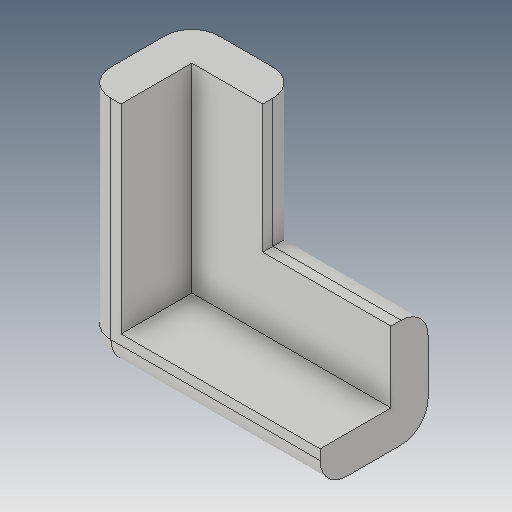
# Autodesk Inventor part: クッション
Saved by Autodesk Inventor 2020.3 (Build 243373000, 373)
## iProperties
Part Number: クッション
Material: 一般
Document SubType Name: Modeling
Designer: highs
Density: 1 g/cm^3
Appearance: 既定
Description: https://jp.misumi-ec.com/vona2/detail/223006733679/?KWSearch=%e8%a7%92%e3%82%af%e3%83%83%e3%82%b7%e3%83%a7%e3%83%b3&searchFlow=results2products
Stock Number: 数と色はナビトンに準拠
Author: highs
Revision Number: 6個使っている？
Autodesk Inventor part; units mm, degrees
ref_plane "YZ Plane" through (0, 0, 0) normal (1, 0, 0) x (0, 1, 0)
ref_plane "XZ Plane" through (0, 0, 0) normal (0, 1, 0) x (-1, 0, 0)
ref_plane "XY Plane" through (0, 0, 0) normal (0, 0, 1) x (1, 0, 0)
sketch "スケッチ1" plane through (0, 0, 0) normal (0, 0, 1) x (1, 0, 0)
  line L0 (0, 0) -> (70, 0)
  line L1 (70, 0) -> (70, 32)
  line L2 (70, 32) -> (32, 32)
  line L3 (32, 32) -> (32, 70)
  line L4 (32, 70) -> (0, 70)
  line L5 (0, 70) -> (0, 0)
  dimension "d0" = 70
  dimension "d1" = 70
  dimension "d3" = 32
  dimension "d4" = 32
  constraints: 12 end point, 5 perpendicular, 1 horizontal
  measures "d0" distance of L4.end L0.start
  measures "d1" distance of L0.start L0.end
  measures "d3" distance of L3.end L4.end
  measures "d4" distance of L0.end L1.end
extrude "押し出し1" add sketch "スケッチ1" along normal blind 32
sketch "スケッチ2" plane through (0, 0, 32) normal (0, 0, 1) x (1, 0, 0)
  line L0 (11, 11) -> (70, 11)
  line L1 (70, 11) -> (70, 70)
  line L2 (70, 70) -> (11, 70)
  line L3 (11, 70) -> (11, 11)
  line L4 (32, 70) -> (0, 70) projected
  line L5 (70, 0) -> (70, 32) projected
  line L6 (32, 32) -> (32, 70) projected
  line L7 (70, 32) -> (32, 32) projected
  point P0 (0, 0)
  dimension "d11" = 21
  dimension "d12" = 21
  constraints: 8 end point, 2 collinear, 2 parallel, 1 horizontal, 1 perpendicular
  measures "d11" distance between parallel lines of L6 L3
  measures "d12" distance between parallel lines of L7 L0
extrude "押し出し2" cut sketch "スケッチ2" against normal blind 21
fillet "フィレット1" radius 8 7 edges at (32, 51, 0) (51, 32, 0) (0, 35, 0) (35, 0, 0) (0, 0, 16) (0, 35, 32) (35, 0, 32)
